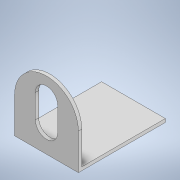
# Autodesk Inventor part: LBracket
Saved by Autodesk Inventor 2022.2 (Build 262287010, 287A)
## iProperties
Created: 2022-03-28
Part Number: LBracket
Material: Generic
Document SubType Name: Modeling
Designer: Santiago Larraín
Density: 1 g/cm^3
Appearance: Default
Author: Santiago Larraín
Autodesk Inventor part; units mm, degrees
ref_plane "YZ Plane" through (0, 0, 0) normal (1, 0, 0) x (0, 1, 0)
ref_plane "XZ Plane" through (0, 0, 0) normal (0, 1, 0) x (-1, 0, 0)
ref_plane "XY Plane" through (0, 0, 0) normal (0, 0, 1) x (1, 0, 0)
sketch "Sketch1" plane through (0, 0, 0) normal (0, 1, 0) x (-1, 0, 0)
  line L0 (-18.8, 25.65) -> (-18.8, -25.65)
  line L1 (-18.8, -25.65) -> (18.8, -25.65)
  line L2 (18.8, -25.65) -> (18.8, 25.65)
  line L3 (18.8, 25.65) -> (-18.8, 25.65)
  line L4 (-18.8, 25.65) -> (18.8, -25.65) construction
  line L5 (-18.8, -25.65) -> (18.8, 25.65) construction
  point P0 (0, 0)
  dimension "d0" = 51.3
  dimension "d1" = 37.6
  constraints: 12 end point, 2 midpoint, 2 parallel, 1 perpendicular, 1 vertical
  measures "d0" distance of L0.start L0.end
  measures "d1" distance of L1.end L0.end
extrude "Extrusion1" add sketch "Sketch1" along normal blind 2
sketch "Sketch2" plane through (-18.8, 0, 25.65) normal (0, 0, 1) x (1, 0, 0)
  line L0 (37.6, 2) -> (0, 2) projected
  line L1 (0, 2) -> (37.6, 2)
  line L2 (37.6, 2) -> (37.6, 21.19)
  line L3 (0, 21.19) -> (0, 2)
  arc A0 (37.6, 21.19) -> (0, 21.19) centre (18.8, 21.19) ccw
  arc A1 (18.8, 7.667) -> (25.4, 14.267) centre (18.8, 14.267) ccw
  arc A2 (12.2, 14.267) -> (18.8, 7.667) centre (18.8, 14.267) ccw
  arc A3 (25.4, 28.267) -> (18.8, 34.867) centre (18.8, 28.267) ccw
  arc A4 (18.8, 34.867) -> (12.2, 28.267) centre (18.8, 28.267) ccw
  line L4 (12.2, 28.267) -> (12.2, 14.267)
  line L5 (25.4, 28.267) -> (25.4, 14.267)
  point P0 (18.8, 0)
  dimension "d5" = 7.667
  dimension "d6" = 27.2
  constraints: 13 point on circle, 10 end point, 5 centre point, 3 equal length, 2 coincident, 2 concentric, 1 perpendicular, 1 vertical
  measures "d5" distance of point (18.8, 0) A1.start
  measures "d6" distance of A1.start A3.end
extrude "Extrusion2" add sketch "Sketch2" against normal blind 2
body "Solid1"
